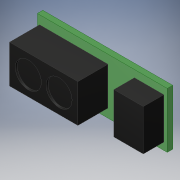
# Autodesk Inventor part: IR Sensor
Saved by Autodesk Inventor 2019.4 (Build 234330000, 330)
## iProperties
Created: 2020-09-04
Part Number: IR Sensor
Material: Generic
Document SubType Name: Modeling
Designer: Mike Angus
Density: 1 g/cm^3
Appearance: Smooth - Dark Forest Green
Author: Mike Angus
Autodesk Inventor part; units mm, degrees
ref_plane "YZ Plane" through (0, 0, 0) normal (1, 0, 0) x (0, 1, 0)
ref_plane "XZ Plane" through (0, 0, 0) normal (0, 1, 0) x (-1, 0, 0)
ref_plane "XY Plane" through (0, 0, 0) normal (0, 0, 1) x (1, 0, 0)
sketch "Sketch1" plane through (0, 0, 0) normal (0, 0, 1) x (1, 0, 0)
  line L0 (0, 4.05) -> (19, 4.05)
  line L1 (19, 4.05) -> (19, -4.05)
  line L2 (19, -4.05) -> (0, -4.05)
  line L3 (0, -4.05) -> (0, 4.05)
  line L4 (0, 4.05) -> (19, -4.05) construction
  line L5 (19, 4.05) -> (0, -4.05) construction
  point P0 (0, 0)
  point P1 (9.5, 0)
  point P2 (0, 0)
  dimension "d0" = 19
  dimension "d1" = 8.1
  constraints: 12 end point, 3 midpoint, 2 parallel, 1 coincident, 1 horizontal, 1 perpendicular
  measures "d0" distance of L0.start L0.end
  measures "d1" distance of L0.end L1.end
extrude "Extrusion1" add sketch "Sketch1" against normal blind 0.8
sketch "Sketch2" plane through (0, 0, 0) normal (0, 0, 1) x (1, 0, 0)
  line L0 (0.33, 2.775) -> (10.33, 2.775)
  line L1 (10.33, 2.775) -> (10.33, -2.775)
  line L2 (10.33, -2.775) -> (0.33, -2.775)
  line L3 (0.33, -2.775) -> (0.33, 2.775)
  line L4 (0.33, 2.775) -> (10.33, -2.775) construction
  line L5 (10.33, 2.775) -> (0.33, -2.775) construction
  line L6 (0, 0) -> (0.33, 0) construction
  line L7 (19, 4.05) -> (19, -4.05) construction
  line L8 (19, 0) -> (18.5, 0) construction
  line L9 (14.2, 3) -> (18.5, 3)
  line L10 (18.5, 3) -> (18.5, -3)
  line L11 (18.5, -3) -> (14.2, -3)
  line L12 (14.2, -3) -> (14.2, 3)
  line L13 (14.2, 3) -> (18.5, -3) construction
  line L14 (18.5, 3) -> (14.2, -3) construction
  point P0 (5.33, 0)
  point P1 (16.35, 0)
  dimension "d4" = 0.33
  dimension "d5" = 5.55
  dimension "d6" = 10
  dimension "d7" = 0.5
  dimension "d8" = 6
  dimension "d9" = 4.3
  constraints: 28 end point, 7 midpoint, 4 horizontal, 4 parallel, 2 perpendicular, 1 coincident
  measures "d4" distance of L6.end L6.start
  measures "d5" distance of L2.end L0.start
  measures "d6" distance of L0.start L0.end
  measures "d7" distance of L8.end L8.start
  measures "d8" distance of L11.end L9.start
  measures "d9" distance of L9.start L9.end
extrude "Extrusion2" add sketch "Sketch2" along normal blind 4.4 separate body contours L0 L1 L2 L3
extrude "Extrusion3" add sketch "Sketch2" along normal blind 3 contours L9 L10 L11 L12 bodies 2
sketch "Sketch3" plane through (0, 0, 4.4) normal (0, 0, 1) x (1, 0, 0)
  line L0 (0.33, 2.775) -> (10.33, 2.775) construction
  line L1 (5.33, 2.775) -> (5.33, -2.775) construction
  line L2 (10.33, -2.775) -> (0.33, -2.775) construction
  line L3 (0.33, 2.775) -> (0.33, -2.775) construction
  line L4 (10.33, -2.775) -> (10.33, 2.775) construction
  line L5 (3.08, 0) -> (7.58, 0) construction
  circle A0 centre (3.08, 0) radius 1.9
  circle A1 centre (7.58, 0) radius 1.9
  point P0 (0, 0)
  point P1 (5.33, 0)
  dimension "d14" = 4.5
  dimension "d15" = 3.8
  dimension "d16" = 3.8
  constraints: 4 end point, 4 midpoint, 2 centre point, 2 coincident, 1 horizontal
  measures "d14" distance of L5.start L5.end
  measures "d15" diameter of A0
  measures "d16" diameter of A1
extrude "Extrusion4" cut sketch "Sketch3" against normal blind 0.3 bodies 2
equation "\"d0\" = ir_length"
equation "\"d1\" = ir_width"
equation "\"d2\" = ir_depth"
equation "\"d4\" = ir_blockOffset"
equation "\"d5\" = ir_blockWidth"
equation "\"d6\" = ir_blockLength"
equation "\"d7\" = ir_connOffset"
equation "\"d8\" = ir_connWidth"
equation "\"d9\" = ir_connLength"
equation "\"d10\" = ir_blockDepth"
equation "\"d12\" = ir_connDepth"
equation "\"d14\" = ir_ledSpacing"
equation "\"d15\" = ir_ledDiam"
equation "\"d16\" = ir_ledDiam"
equation "\"d17\" = ir_ledDepth"
equation "\"ir_length\" = 19"
equation "\"ir_width\" = 8.1"
equation "\"ir_depth\" = 0.8"
equation "\"ir_blockLength\" = 10"
equation "\"ir_blockWidth\" = 5.55"
equation "\"ir_blockDepth\" = 4.4"
equation "\"ir_connWidth\" = 6"
equation "\"ir_connLength\" = 4.3"
equation "\"ir_connDepth\" = 3"
equation "\"ir_blockOffset\" = 0.33"
equation "\"ir_connOffset\" = 0.5"
equation "\"ir_ledDiam\" = 3.8"
equation "\"ir_ledSpacing\" = 4.5"
equation "\"ir_ledDepth\" = 0.3"
body "Solid1"
body "Solid2"
